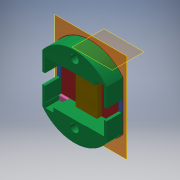
# Autodesk Inventor part: KEEPOUT_BOTTOM
Saved by Autodesk Inventor 2016 (Build 200138000, 138)
## iProperties
Created: 2016-09-29
Part Number: KEEPOUT_BOTTOM
Material: Generic
Document SubType Name: Modeling
Designer: benja
Density: 1 g/cm^3
Appearance: Default
Author: benja
Autodesk Inventor part; units mm, degrees
ref_plane "YZ Plane" through (0, 0, 0) normal (1, 0, 0) x (0, 1, 0)
ref_plane "XZ Plane" through (0, 0, 0) normal (0, 1, 0) x (-1, 0, 0)
ref_plane "XY Plane" through (0, 0, 0) normal (0, 0, 1) x (1, 0, 0)
ref_plane "Work Plane1" through (0, 40.5, -6.5875) normal (0, 1, 0) x (1, 0, 0)
ref_plane "Work Plane2" through (0, 0, 0) normal (0, 0, 1) x (1, 0, 0)
sketch "KEEPOUT_BOT_0.1MM_S" plane through (0, 0, 0) normal (0, 0, 1) x (1, 0, 0)
  circle A0 centre (0, -25) radius 1.75 projected
  circle A1 centre (-14, -14) radius 1.75 projected
  circle A2 centre (22, -14) radius 1.75 projected
  circle A3 centre (14, 14) radius 1.75 projected
  circle A4 centre (-22, 14) radius 1.75 projected
  circle A5 centre (0, 30) radius 1.75 projected
  line L0 (-30, 22.5) -> (-30, -22.5) projected
  arc A6 (-30, -22.5) -> (30, -22.5) centre (0, 0) ccw projected
  line L1 (30, -22.5) -> (30, 22.5) projected
  arc A7 (30, 22.5) -> (-30, 22.5) centre (0, 0) ccw projected
  circle A8 centre (0, -25) radius 3.75 projected
  circle A9 centre (0, 30) radius 3.75 projected
  circle A10 centre (-22, 14) radius 1.75 projected
  circle A11 centre (-14, -14) radius 1.75 projected
  line L2 (-18.5, 11.6278) -> (-26.55, 11.6278) projected
  arc A12 (-16.5, 9.6278) -> (-18.5, 11.6278) centre (-18.5, 9.6278) ccw projected
  line L3 (-16.5, -17) -> (-16.5, 9.6278) projected
  arc A13 (-16.7679, -18) -> (-16.5, -17) centre (-18.5, -17) ccw projected
  line L4 (-16.7679, -18) -> (-12.5, -18) projected
  arc A14 (-12.5, -18) -> (-10.5, -16) centre (-12.5, -16) ccw projected
  line L5 (-10.5, 15.6278) -> (-10.5, -16) projected
  arc A15 (-10.5, 15.6278) -> (-12.5, 17.6278) centre (-12.5, 15.6278) ccw projected
  line L6 (-24.55, 17.6278) -> (-12.5, 17.6278) projected
  arc A16 (-24.55, 17.6278) -> (-26.55, 15.6278) centre (-24.55, 15.6278) ccw projected
  line L7 (-26.55, 11.6278) -> (-26.55, 15.6278) projected
  circle A17 centre (22, -14) radius 1.75 projected
  circle A18 centre (14, 14) radius 1.75 projected
  line L8 (18.5, -11.6278) -> (26.55, -11.6278) projected
  arc A19 (16.5, -9.6278) -> (18.5, -11.6278) centre (18.5, -9.6278) ccw projected
  line L9 (16.5, 17) -> (16.5, -9.6278) projected
  arc A20 (16.7679, 18) -> (16.5, 17) centre (18.5, 17) ccw projected
  line L10 (16.7679, 18) -> (12.5, 18) projected
  arc A21 (12.5, 18) -> (10.5, 16) centre (12.5, 16) ccw projected
  line L11 (10.5, -15.6278) -> (10.5, 16) projected
  arc A22 (10.5, -15.6278) -> (12.5, -17.6278) centre (12.5, -15.6278) ccw projected
  line L12 (24.55, -17.6278) -> (12.5, -17.6278) projected
  arc A23 (24.55, -17.6278) -> (26.55, -15.6278) centre (24.55, -15.6278) ccw projected
  line L13 (26.55, -11.6278) -> (26.55, -15.6278) projected
  line L14 (23.1, 22.02) -> (24.3, 22.02) projected
  line L15 (26.55, -15.6278) -> (26.55, 4.9922) projected
  line L16 (-23.1, -22.02) -> (-24.3, -22.02) projected
  line L17 (-26.55, -11.0422) -> (-26.55, -17) projected
  line L18 (26.7562, -18.1278) -> (10, -18.1278)
  line L19 (10, -18.1278) -> (10, 18.5)
  line L20 (10, 18.5) -> (27.05, 18.5)
  line L21 (27.05, 18.5) -> (27.05, -18.1278)
  line L22 (27.05, -18.1278) -> (26.7562, -18.1278)
  line L23 (-10, -18.5) -> (-27.05, -18.5)
  line L24 (-27.05, -18.5) -> (-27.05, 18.1278)
  line L25 (-27.05, 18.1278) -> (-10, 18.1278)
  line L26 (-10, 18.1278) -> (-10, -18.5)
  arc A24 (-29.5, -22.3327) -> (29.5, -22.3327) centre (0, 0) ccw
  line L27 (-29.5, -22.3327) -> (-29.5, 22.3327)
  arc A25 (29.5, 22.3327) -> (-29.5, 22.3327) centre (0, 0) ccw
  line L28 (29.5, 22.3327) -> (29.5, -22.3327)
  point P0 (0, 0)
  dimension "d0" = 0.5
  dimension "d1" = 0.5
  dimension "d2" = 0.5
  dimension "d3" = 0.5
  dimension "d4" = 0.5
  dimension "d5" = 0.5
  dimension "d6" = 0.5
  dimension "d7" = 0.5
  dimension "d12" = 0.5
  constraints: 22 end point, 4 perpendicular, 4 point on circle, 3 parallel, 2 centre point, 2 horizontal, 1 point on line, 3 other
  measures "d0" distance between parallel lines of L19 L11
  measures "d1" distance between parallel lines of L18 L12
  measures "d2" distance between parallel lines of L15 L21
  measures "d3" distance between parallel lines of L10 L20
  measures "d4" distance between parallel lines of L4 L23
  measures "d5" distance between parallel lines of L5 L26
  measures "d6" distance between parallel lines of L6 L25
  measures "d7" distance between parallel lines of L7 L24
  measures "d12" distance between parallel lines of L28 L1
extrude "KEEPUT_BOT_0.1MM" add sketch "KEEPOUT_BOT_0.1MM_S" along normal blind 0.1 contours A0 | A1 | A2 | A3 | A4 | A5 | A7 L1 A6 L0 | A8 | A9 | L2 L7 A16 L6 A15 L5 A14 L4 A13 L3 A12 | L8 L13 A23 L12 A22 L11 A21 L10 A20 L9 A19 | L18 L19 L20 L21 L22 | L23 L24 L25 L26
ref_plane "Work Plane3" through (0, 0, 0) normal (0, 0, 1) x (1, 0, 0)
sketch "KEEPOUT_BOT_1.5MM_S" plane through (0, 0, 0) normal (0, 0, 1) x (1, 0, 0)
  line L0 (10, -18.1278) -> (27.05, -18.1278)
  line L1 (27.05, -18.1278) -> (27.05, 18.5)
  line L2 (27.05, 18.5) -> (10, 18.5)
  line L3 (10, 18.5) -> (10, -18.1278)
  line L4 (21.9, 22.02) -> (23.1, 22.02)
  line L5 (19.8, 18.35) -> (19.8, 20.35)
  line L6 (27.05, 18.5) -> (19.3, 18.5)
  line L7 (19.3, 18.5) -> (19.3, 22.52)
  line L8 (19.3, 22.52) -> (27.05, 22.52)
  line L9 (27.05, 22.52) -> (27.05, 18.5)
  line L10 (27.4, -5) -> (30.4, -5)
  line L11 (27.4, 5) -> (30.4, 5)
  line L12 (-29.5, -22.3327) -> (-29.5, 22.3327)
  arc A0 (29.5, 22.3327) -> (-29.5, 22.3327) centre (0, 0) ccw
  line L13 (29.5, 22.3327) -> (29.5, -22.3327)
  arc A1 (-29.5, -22.3327) -> (29.5, -22.3327) centre (0, 0) ccw
  line L14 (-30, 22.5) -> (-30, -22.5)
  arc A2 (-30, -22.5) -> (30, -22.5) centre (0, 0) ccw
  line L15 (30, -22.5) -> (30, 22.5)
  arc A3 (30, 22.5) -> (-30, 22.5) centre (0, 0) ccw
  line L16 (29.5, 22.3327) -> (29.5, -22.3327)
  line L17 (27.05, 18.5) -> (27.05, -18.1278)
  line L18 (29.5, 5) -> (27.05, 5)
  line L19 (27.05, 5) -> (27.05, -5)
  line L20 (27.05, -5) -> (29.5, -5)
  line L21 (29.5, -5) -> (29.5, 5)
  line L22 (-27.05, -18.5) -> (-10, -18.5)
  line L23 (-10, -18.5) -> (-10, 18.1278)
  line L24 (-10, 18.1278) -> (-27.05, 18.1278)
  line L25 (-27.05, 18.1278) -> (-27.05, -18.5)
  line L26 (-27.4, 5) -> (-30.4, 5)
  line L27 (-27.4, -5) -> (-30.4, -5)
  line L28 (-29.5, 22.3327) -> (-29.5, -22.3327)
  line L29 (-29.5, -5) -> (-27.05, -5)
  line L30 (-27.05, -5) -> (-27.05, 5)
  line L31 (-27.05, 5) -> (-29.5, 5)
  line L32 (-29.5, 5) -> (-29.5, -5)
  line L33 (-23.1, -22.02) -> (-24.3, -22.02)
  line L34 (-19.8, -10.37) -> (-19.8, -19.37)
  line L35 (-10, -18.5) -> (-27.05, -18.5)
  line L36 (-27.05, -18.5) -> (-19.8, -18.5)
  line L37 (-19.8, -18.5) -> (-19.8, -22.02)
  line L38 (-19.8, -22.02) -> (-27.05, -22.02)
  line L39 (-27.05, -22.02) -> (-27.05, -18.5)
  point P0 (0, 0)
extrude "KEEPOUT_BOT_1.5MM" add sketch "KEEPOUT_BOT_1.5MM_S" along normal blind 1.5 separate body contours L1 L18 L11 L13 L10 L20 | L12 L26 L31 L25 L29 L27
ref_plane "Work Plane4" through (0, 0, 0) normal (0, 0, 1) x (1, 0, 0)
sketch "KEEPOUT_BOT_2.5MM_S" plane through (0, 0, 0) normal (0, 0, 1) x (1, 0, 0)
  line L0 (23.1, 22.02) -> (24.3, 22.02) projected
  line L1 (19.8, 10.37) -> (19.8, 19.37) projected
  line L2 (26.4, 10.37) -> (26.4, 19.37) projected
  line L3 (27.05, 18.5) -> (10, 18.5) projected
  line L4 (19.3, 18.5) -> (26.9, 18.5)
  line L5 (26.9, 18.5) -> (26.9, 22.52)
  line L6 (26.9, 22.52) -> (19.3, 22.52)
  line L7 (19.3, 22.52) -> (19.3, 18.5)
  line L8 (-23.1, -22.02) -> (-24.3, -22.02) projected
  line L9 (-19.8, -20.35) -> (-19.8, -10.37) projected
  line L10 (-26.4, -10.37) -> (-26.4, -19.37) projected
  line L11 (-27.05, -18.5) -> (-10, -18.5) projected
  line L12 (-26.7119, -18.5) -> (-19.2922, -18.5)
  line L13 (-19.2922, -18.5) -> (-19.2922, -22.4447)
  line L14 (-19.2922, -22.4447) -> (-26.7119, -22.4447)
  line L15 (-26.7119, -22.4447) -> (-26.7119, -18.5)
  point P0 (0, 0)
  dimension "d15" = 0.5
  dimension "d16" = 0.5
  dimension "d17" = 0.5
  constraints: 16 end point, 4 parallel, 2 horizontal, 2 perpendicular, 2 point on line
  measures "d15" distance between parallel lines of L6 L0
  measures "d16" distance between parallel lines of L7 L1
  measures "d17" distance between parallel lines of L2 L5
extrude "KEEPOUT_BOT_2.5MM" add sketch "KEEPOUT_BOT_2.5MM_S" along normal blind 2.5 separate body
ref_plane "Work Plane5" through (0, 0, 0) normal (0, 0, 1) x (1, 0, 0)
sketch "KEEPOUT_BOT_4MM_s" plane through (0, 0, 0) normal (0, 0, 1) x (1, 0, 0)
  circle A0 centre (22, -14) radius 1.75 projected
  circle A1 centre (14, 14) radius 1.75 projected
  line L0 (18.5, -11.6278) -> (26.55, -11.6278) projected
  arc A2 (16.5, -9.6278) -> (18.5, -11.6278) centre (18.5, -9.6278) ccw projected
  line L1 (16.5, 17) -> (16.5, -9.6278) projected
  arc A3 (16.7679, 18) -> (16.5, 17) centre (18.5, 17) ccw projected
  line L2 (16.7679, 18) -> (12.5, 18) projected
  arc A4 (12.5, 18) -> (10.5, 16) centre (12.5, 16) ccw projected
  line L3 (10.5, -15.6278) -> (10.5, 16) projected
  arc A5 (10.5, -15.6278) -> (12.5, -17.6278) centre (12.5, -15.6278) ccw projected
  line L4 (24.55, -17.6278) -> (12.5, -17.6278) projected
  arc A6 (24.55, -17.6278) -> (26.55, -15.6278) centre (24.55, -15.6278) ccw projected
  line L5 (26.55, -11.6278) -> (26.55, -15.6278) projected
  circle A7 centre (-22, 14) radius 1.75 projected
  circle A8 centre (-14, -14) radius 1.75 projected
  line L6 (-18.5, 11.6278) -> (-26.55, 11.6278) projected
  arc A9 (-16.5, 9.6278) -> (-18.5, 11.6278) centre (-18.5, 9.6278) ccw projected
  line L7 (-16.5, -17) -> (-16.5, 9.6278) projected
  arc A10 (-16.7679, -18) -> (-16.5, -17) centre (-18.5, -17) ccw projected
  line L8 (-16.7679, -18) -> (-12.5, -18) projected
  arc A11 (-12.5, -18) -> (-10.5, -16) centre (-12.5, -16) ccw projected
  line L9 (-10.5, 15.6278) -> (-10.5, -16) projected
  arc A12 (-10.5, 15.6278) -> (-12.5, 17.6278) centre (-12.5, 15.6278) ccw projected
  line L10 (-24.55, 17.6278) -> (-12.5, 17.6278) projected
  arc A13 (-24.55, 17.6278) -> (-26.55, 15.6278) centre (-24.55, 15.6278) ccw projected
  line L11 (-26.55, 11.6278) -> (-26.55, 15.6278) projected
  line L12 (10, -18.5) -> (-10, -18.5)
  line L13 (-10, -18.5) -> (-10, 18.5)
  line L14 (-10, 18.5) -> (10, 18.5)
  line L15 (10, 18.5) -> (10, -18.5)
  point P0 (0, 0)
  constraints: 8 end point, 2 coincident, 2 parallel, 1 horizontal, 1 perpendicular
extrude "KEEPOUT_BOT_4MM" add sketch "KEEPOUT_BOT_4MM_s" along normal blind 4 contours L12 L13 L14 L15 bodies 1
ref_plane "Work Plane6" through (0, 0, 0) normal (0, 0, 1) x (1, 0, 0)
sketch "KEEPOUT_BOT_15MM_S" plane through (0, 0, 0) normal (0, 0, 1) x (1, 0, 0)
  arc A0 (-29.5, -22.3327) -> (29.5, -22.3327) centre (0, 0) ccw projected
  line L0 (29.5, 22.3327) -> (29.5, -22.3327) projected
  line L1 (27.05, -5) -> (29.5, -5) projected
  line L2 (27.05, -18.1278) -> (27.05, 18.5) projected
  line L3 (10, -18.1278) -> (27.05, -18.1278) projected
  line L4 (-10, -18.5) -> (10, -18.5) projected
  line L5 (-27.05, -18.5) -> (-10, -18.5) projected
  line L6 (-19.2922, -18.5) -> (-19.2922, -22.4447) projected
  line L7 (-19.2922, -22.4447) -> (-26.7119, -22.4447) projected
  line L8 (-26.7119, -22.4447) -> (-26.7119, -18.5) projected
  line L9 (-27.05, 18.1278) -> (-27.05, -18.5) projected
  line L10 (-29.5, -5) -> (-27.05, -5) projected
  line L11 (-29.5, -22.3327) -> (-29.5, 22.3327) projected
  line L12 (-27.05, 5) -> (-29.5, 5) projected
  line L13 (-10, 18.1278) -> (-27.05, 18.1278) projected
  line L14 (-10, 18.1278) -> (-10, 18.5) projected
  line L15 (-10, 18.5) -> (27.05, 18.5) projected
  arc A1 (29.5, 22.3327) -> (-29.5, 22.3327) centre (0, 0) ccw projected
  circle A2 centre (0, -25) radius 3.75 projected
  circle A3 centre (0, 30) radius 3.75 projected
  line L16 (29.5, 5) -> (27.05, 5) projected
  line L17 (19.3, 18.5) -> (26.9, 18.5) projected
  line L18 (26.9, 18.5) -> (26.9, 22.52) projected
  line L19 (26.9, 22.52) -> (19.3, 22.52) projected
  line L20 (19.3, 22.52) -> (19.3, 18.5) projected
  line L21 (10, -18.1278) -> (10, -18.5) projected
  line L22 (-24.93, -13.25) -> (-24.93, -1.6425) projected
  line L23 (-29.5, 22.3327) -> (-29.5, -22.3327) projected
  point P0 (0, 0)
extrude "KEEPOUT_BOT_15MM" add sketch "KEEPOUT_BOT_15MM_S" along normal blind 15 separate body contours L11 L10 L9 L5 L8 L7 L6 L4 L21 L3 L2 L1 L0 A0 | L11 A1 L0 L16 L2 L15 L18 L19 L20 L14 L13 L9 L12
equation "\"d1\" = d0"
equation "\"d2\" = d1"
equation "\"d3\" = d0"
equation "\"d4\" = d1"
equation "\"d5\" = d1"
equation "\"d6\" = d3"
equation "\"d7\" = d3"
equation "\"d16\" = d15"
equation "\"d17\" = d15"
equation "\"d11\" = d10"
equation "\"d10\" = 0.5"
body "Solid1"
body "Solid2"
body "Solid3"
body "Solid4"
